Autodesk Fusion 360 part; units mm, degrees
note: some values were not read from the file. Chosen so that the rebuilt part matches the saved one: which face or edge a step refers to; how an offset face is resized; the sign of a taper; which pieces of a blend or face edit are solid. Set by a fixed rule: which sketch regions a step uses.
(part 2 of 2)
Autodesk Fusion 360 part; units mm, degrees
sketch "Sketch1" plane through (0, 0, 0) normal (0, 1, 0) x (1, 0, 0)
  line L0 (2.75, -2.75) -> (5.75, -2.75)
  arc A0 (5.75, -2.75) -> (5.75, 2.75) centre (5.75, 0) ccw
  line L1 (5.75, 2.75) -> (2.75, 2.75)
  arc A1 (2.75, 2.75) -> (2.75, -2.75) centre (2.75, 0) ccw
  line L2 (0, 0) -> (8.5, 0) construction
  arc A2 (2.75, 4.75) -> (2.75, -4.75) centre (2.75, 0) ccw
  line L3 (2.75, -4.75) -> (5.75, -4.75)
  arc A3 (5.75, -4.75) -> (5.75, 4.75) centre (5.75, 0) ccw
  line L4 (5.75, 4.75) -> (2.75, 4.75)
  line L5 (10.5, 0) -> (10.5, 23)
  line L6 (10.5, 23) -> (-2, 23)
  line L7 (-2, 23) -> (-2, 0)
  dimension "d1" = 5.5
  dimension "d2" = 8.5
  dimension "d3" = 2
  dimension "d4" = 23
  constraint tangent L0 A0
  constraint tangent A0 L1
  constraint parallel L0 L1
  constraint tangent L1 A1
  constraint tangent L0 A1
  constraint midpoint A1 L2.start
  constraint midpoint A0 L2.end
  constraint horizontal L2
  constraint coincident L2.start origin
  constraint vertical L5
  constraint horizontal L6
  constraint vertical L7
  constraint midpoint A2 L7.end
  measures "d1" diameter of A0
  measures "d2" distance of L2.start L2.end
  measures "d4" distance of L5.start L5.end
extrude "Extrude1" add sketch "Sketch1" along normal blind 7
sketch "Sketch2" plane through (0, 0, -23) normal (0, 0, -1) x (1, 0, 0)
  line L0 (10.5, 0) -> (-2, 0)
  line L1 (-2, 0) -> (-2, -7)
  line L2 (-2, -7) -> (10.5, -7)
  line L3 (10.5, -7) -> (10.5, 0)
  line L4 (-2, 0) -> (10.5, 0)
  line L5 (10.5, 0) -> (10.5, 12)
  line L6 (10.5, 12) -> (-2, 12)
  line L7 (-2, 12) -> (-2, 0)
  circle A0 centre (4.25, 7) radius 2.25
  dimension "d7" = 12.5
  dimension "d8" = 12
  dimension "d9" = 12.5
  dimension "d10" = 4.5
  dimension "d11" = 7
  constraint horizontal L4
  constraint vertical L5
  constraint horizontal L6
  constraint vertical L7
  constraint coincident L0.end L1.start
  measures "d7" distance of L0.end L0.start
  measures "d8" distance of L0.end L6.end
  measures "d9" distance of L0.start L0.end
  measures "d10" diameter of A0
  measures "d11" distance of L4 A0.centre
extrude "Extrude2" add sketch "Sketch2" against normal blind 3 contours L0 L4 L5 L6 L7
chamfer "Chamfer1" distance 2 angle 45 1 edges at (4.25, 0, -20)
other "Screw1"
component "drzalo za oba kabla v5" placed x (1, 0, 0) y (0, 1, 0) z (0, 0, 1) at (0, 0, 0)
equation "d7 = d9"
equation "d11 = d8 / 2 + 1 mm"
